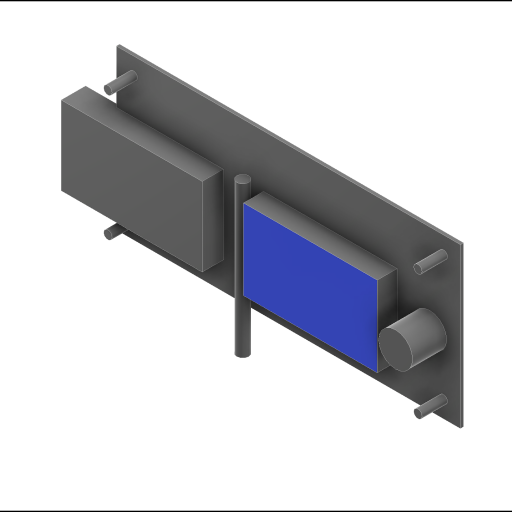
# Autodesk Inventor part: Circuit Board Mockup
Saved by Autodesk Inventor 2023 (Build 270158000, 158)
## iProperties
Created: 2022-11-05
Part Number: Circuit Board Mockup
Material: Generic
Document SubType Name: Modeling
Designer: kamer
Density: 1 g/cm^3
Appearance: Smooth - Black
Mass: 287.17 g
Surface Area: 830.013 cm^2
Volume: 287.17 cm^3
Author: kamer
Autodesk Inventor part; units mm, degrees
ref_plane "YZ Plane" through (0, 0, 0) normal (1, 0, 0) x (0, 1, 0)
ref_plane "XZ Plane" through (0, 0, 0) normal (0, 1, 0) x (-1, 0, 0)
ref_plane "XY Plane" through (0, 0, 0) normal (0, 0, 1) x (1, 0, 0)
sketch "Sketch1" plane through (0, 0, 0) normal (0, 0, 1) x (1, 0, 0)
  line L0 (0, 0) -> (257.175, 0)
  line L1 (257.175, 0) -> (257.175, 119.0625)
  line L2 (257.175, 119.0625) -> (0, 119.0625)
  line L3 (0, 119.0625) -> (0, 0)
  dimension "d0" = 257.175
  dimension "d1" = 119.0625
  constraints: 8 end point, 2 parallel, 1 horizontal, 1 perpendicular
  measures "d0" distance of L1.end L2.end
  measures "d1" distance of L0.end L1.end
extrude "Extrusion1" add sketch "Sketch1" along normal blind 2.3813
sketch "Sketch2" plane through (0, 0, 2.3813) normal (0, 0, 1) x (1, 0, 0)
  circle A0 centre (12.7, 106.3625) radius 3.175
  circle A1 centre (244.475, 106.3625) radius 3.175
  circle A2 centre (244.475, 12.7) radius 3.175
  circle A3 centre (12.7, 12.7) radius 3.175
  line L0 (0, 0) -> (257.175, 0) projected
  line L1 (0, 119.0625) -> (0, 0) projected
  line L2 (257.175, 119.0625) -> (0, 119.0625) projected
  line L3 (257.175, 0) -> (257.175, 119.0625) projected
  dimension "d4" = 6.35
  dimension "d5" = 6.35
  dimension "d6" = 6.35
  dimension "d7" = 6.35
  dimension "d8" = 12.7
  dimension "d9" = 12.7
  dimension "d10" = 12.7
  dimension "d11" = 12.7
  dimension "d12" = 12.7
  dimension "d13" = 12.7
  dimension "d14" = 12.7
  dimension "d15" = 12.7
  constraints: 4 centre point
  measures "d4" diameter of A0
  measures "d5" diameter of A1
  measures "d6" diameter of A2
  measures "d7" diameter of A3
  measures "d8" distance from line of L0 A3.centre
  measures "d9" distance from line of L1 A3.centre
  measures "d10" distance from line of L2 A0.centre
  measures "d11" distance from line of L1 A0.centre
  measures "d12" distance from line of L2 A1.centre
  measures "d13" distance from line of A1.centre L3
  measures "d14" distance from line of L3 A2.centre
  measures "d15" distance from line of A2.centre L0
extrude "Clearance Distance" add sketch "Sketch2" along normal blind 19.05 contours A0 | A1 | A2 | A3
sketch "Sketch3" plane through (0, 0, 0) normal (-1, 0, 0) x (0, 0, 1)
  line L0 (0, 119.0625) -> (0, 0) projected
  line L1 (0, 20.6375) -> (18.2563, 20.6375)
  line L2 (18.2563, 20.6375) -> (18.2562, 79.375)
  line L3 (18.2562, 79.375) -> (0, 79.375)
  line L4 (0, 79.375) -> (0, 20.6375)
  line L5 (0, 119.0625) -> (2.3813, 119.0625) projected
  point P0 (0, 79.375)
  dimension "d18" = 18.2563
  dimension "d19" = 39.6875
  dimension "d20" = 98.425
  constraints: 8 end point, 2 parallel, 1 horizontal, 1 perpendicular, 1 point on line
  measures "d18" distance between parallel lines of L0 L2
  measures "d19" distance between parallel lines of L5 L3
  measures "d20" distance between parallel lines of L5 L1
extrude "Extrusion3" add sketch "Sketch3" along normal blind 25.4 and the other way blind 80
sketch "Sketch4" plane through (0, 0, 2.3813) normal (0, 0, 1) x (1, 0, 0)
  circle A0 centre (234.1562, 52.3875) radius 12.7
  line L0 (257.175, 119.0625) -> (0, 119.0625) projected
  line L1 (257.175, 0) -> (257.175, 119.0625) projected
  point P0 (0, 0)
  dimension "d25" = 25.4
  dimension "d26" = 66.675
  dimension "d27" = 23.0188
  constraints: 1 centre point
  measures "d25" diameter of A0
  measures "d26" distance from line of L0 A0.centre
  measures "d27" distance from line of L1 A0.centre
extrude "Extrusion4" add sketch "Sketch4" along normal blind 25.4
sketch "Sketch6" plane through (0, 0, 0) normal (0, -1, 0) x (1, 0, 0)
  circle A0 centre (101.6, 9.525) radius 4.4901
  line L0 (0, 0) -> (0, 2.3813) projected
  dimension "d30" = 101.6
  constraints: 1 centre point
  measures "d30" distance from line of L0 A0.centre
extrude "Extrusion5" add sketch "Sketch6" along normal blind 25.4 and the other way blind 87.3125
sketch "Sketch7" plane through (0, 0, 2.3813) normal (0, 0, 1) x (1, 0, 0)
  line L0 (110, 80) -> (210, 80)
  line L1 (210, 80) -> (210, 20)
  line L2 (210, 20) -> (110, 20)
  line L3 (110, 20) -> (110, 80)
  line L4 (0, 119.0625) -> (0, 79.375) projected
  line L5 (0, 20.6375) -> (0, 0) projected
  line L6 (0, 0) -> (257.175, 0) projected
  dimension "d35" = 110
  dimension "d36" = 210
  dimension "d37" = 20
  dimension "d38" = 80
  constraints: 8 end point, 2 parallel, 1 horizontal, 1 perpendicular
  measures "d35" distance between parallel lines of L4 L3
  measures "d36" distance between parallel lines of L5 L1
  measures "d37" distance between parallel lines of L6 L2
  measures "d38" distance between parallel lines of L6 L0
extrude "Extrusion6" add sketch "Sketch7" along normal blind 15
body "Solid1"
